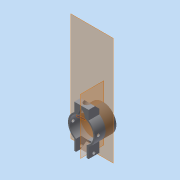
# Autodesk Inventor part: 13_Opentrons_Autofocus_Objectivering_Laser_Cam
Saved by Autodesk Inventor 2019.4 (Build 234330000, 330)
## iProperties
Created: 2020-12-16
Part Number: 13_Opentrons_Autofocus_Objectivering_Laser_Cam
Material: Generic
Document SubType Name: Modeling
Designer: diederichbenedict
Density: 1 g/cm^3
Appearance: Default
Author: diederichbenedict
Autodesk Inventor part; units mm, degrees
ref_plane "YZ Plane" through (0, 0, 0) normal (1, 0, 0) x (0, 1, 0)
ref_plane "XZ Plane" through (0, 0, 0) normal (0, 1, 0) x (-1, 0, 0)
ref_plane "XY Plane" through (0, 0, 0) normal (0, 0, 1) x (1, 0, 0)
ref_plane "Work Plane1" through (0, 0, 0) normal (0, 0, 1) x (1, 0, 0)
sketch "Sketch1" plane through (0, 0, 0) normal (0, 0, 1) x (1, 0, 0)
  circle A0 centre (0.9353, 17.3993) radius 11 projected
  circle A1 centre (0.9353, 17.3993) radius 11.1
  circle A2 centre (0.9353, 17.3993) radius 12.5
  point P0 (0, 0)
  dimension "d0" = 22.2
  dimension "d1" = 25
  constraints: 2 centre point, 2 coincident
  measures "d0" diameter of A1
  measures "d1" diameter of A2
extrude "Extrusion1" add sketch "Sketch1" against normal blind 10 contours A2
sketch "Sketch2" plane through (0.9353, 17.3993, 0) normal (0, 0, 1) x (1, 0, 0)
  circle A0 centre (0, 0) radius 12.5 projected
  circle A1 centre (0, 0) radius 11 construction
  ellipse E0 centre (0, 9.932) end of major axis (3, 9.932) minor radius 1.7207 construction
  ellipse E1 centre (0, -15.992) end of major axis (-4.2, -15.992) minor radius 2.409 construction
  circle A2 centre (0, 0) radius 11.1 projected
  line L0 (-6.6479, 19.2015) -> (6.6479, 19.2015)
  line L1 (6.6479, 19.2015) -> (6.6479, 10.5856)
  line L2 (-6.6479, 10.5856) -> (-6.6479, 19.2015)
  line L3 (-6.6479, 19.2015) -> (9.489, 5.7592) construction
  line L4 (6.6479, 19.2015) -> (-6.2726, 8.4385) construction
  line L5 (9.489, 5.7592) -> (9.3718, 5.7592) construction
  line L6 (-7.0563, 8.4385) -> (-6.2726, 8.4385) construction
  line L7 (-6.6479, -20.4673) -> (6.6479, -20.4673)
  line L8 (6.6479, -20.4673) -> (6.6479, -10.5856)
  line L9 (-6.6479, -10.5856) -> (-6.6479, -20.4673)
  line L10 (-6.6479, -20.4673) -> (6.6479, -10.5856) construction
  line L11 (6.6479, -20.4673) -> (-6.6479, -10.5856) construction
  line L12 (3.3398, -10.5856) -> (2.9907, -10.5856)
  line L13 (-2.9907, -10.5856) -> (-3.3398, -10.5856)
  point P0 (-0.9353, -17.3993)
  point P1 (0, 13.6637)
  point P2 (0, -15.5265)
  constraints: 28 end point, 11 point on circle, 6 parallel, 2 collinear, 2 horizontal, 2 midpoint, 2 perpendicular, 2 point on line, 1 coincident, 2 other
extrude "Extrusion3" add sketch "Sketch2" along normal blind 10
ref_plane "Work Plane2" through (-0.8941, 25.9676, 8.5979) normal (0, -0.819152, 0.5735764) x (0.7925374, -0.3497803, -0.499538)
ref_plane "Work Plane3" through (0.9353, -3.0679, 0) normal (1, 0, 0) x (0, 0, -1)
sketch "Sketch3" plane through (0.9353, -3.0679, 0) normal (1, 0, 0) x (0, 0, -1)
  line L0 (-7.6942, -1.3824) -> (-0.3218, 3.7798) projected
  line L1 (-9.1586, -2.4078) -> (-0.3397, 3.7672)
  line L2 (-0.3397, 3.7672) -> (-9.6168, 17.0163)
  line L3 (-9.6168, 17.0163) -> (-18.4357, 10.8412)
  line L4 (-18.4357, 10.8412) -> (-9.1586, -2.4078)
  line L5 (-9.1586, -2.4078) -> (-0.3397, 3.7672)
  line L6 (-0.3397, 3.7672) -> (-9.1586, -2.4078)
  line L7 (-0.3218, 3.7798) -> (-1.4689, 5.4181) construction
  line L8 (-0.3218, 3.7798) -> (-1.4689, 5.4181) construction
  line L9 (-7.6942, -1.3824) -> (-8.8413, 0.2559) construction
  line L10 (-7.6942, -1.3824) -> (-8.8413, 0.2559) construction
  point P0 (0, 3.0679)
  constraints: 12 end point, 4 equal length, 2 coincident, 1 perpendicular, 1 point on line, 5 other
extrude "Extrusion4" cut sketch "Sketch3" along normal mid plane 10
sketch "Sketch4" plane through (-0.8941, 25.9676, 8.5979) normal (0, -0.819152, 0.5735764) x (0.7925374, -0.3497803, -0.499538)
  circle A0 centre (0, 3) radius 3 projected
  circle A1 centre (0, 3) radius 3.15
  point P0 (14.0866, -16.841)
  dimension "d11" = 6.3
  constraints: 1 centre point, 1 coincident
  measures "d11" diameter of A1
extrude "Extrusion5" cut sketch "Sketch4" against normal through all contours A0 | A1
chamfer "Chamfer1" distance 4 angle 45 1 edges at (0.9353, 36.6008, 0)
sketch "Sketch5" plane through (0.9353, -3.0679, 0) normal (1, 0, 0) x (0, 0, -1)
  line L0 (10, 7.9673) -> (10, 32.9673) projected
  line L1 (0, 9.8817) -> (0, 9.8817) projected
  line L2 (0, 9.8817) -> (-10, 9.8817) projected
  line L3 (-10, 31.0529) -> (-10, 9.8817) projected
  line L4 (0, 31.0529) -> (-10, 31.0529) projected
  line L5 (0, 31.0529) -> (0, 31.0529) projected
  line L6 (0, 31.0529) -> (-10, 31.0529) projected
  line L7 (-10, 9.8817) -> (-10, 31.0529) projected
  line L8 (0, 9.8817) -> (-10, 9.8817) projected
  circle A0 centre (-6.4895, 20.4673) radius 1.45
  point P0 (0, 3.0679)
  dimension "d17" = 2.9
  constraints: 1 centre point
  measures "d17" diameter of A0
extrude "Extrusion6" cut sketch "Sketch5" along normal through all both and the other way through all
sketch "Sketch6" plane through (-5.7126, -3.0679, 0) normal (-1, 0, 0) x (0, 0, 1)
  line L0 (7.6942, -1.3824) -> (0.3218, 3.7798) projected
  line L1 (7.6942, -1.3824) -> (0.3218, 3.7798) projected
  line L2 (7.6942, -1.3824) -> (8.8413, 0.2559) projected
  line L3 (1.4689, 5.4181) -> (8.8413, 0.2559) projected
  line L4 (0.3218, 3.7798) -> (1.4689, 5.4181) projected
  circle A0 centre (4.8882, 2.4558) radius 1.45
  point P0 (0, 3.0679)
  dimension "d20" = 2.9
  constraints: 1 centre point
  measures "d20" diameter of A0
extrude "Extrusion7" cut sketch "Sketch6" against normal through all contours A0 L3 | L3 A0
pattern_circular "Circular Pattern1" count 2 over 30 about axis through (0.9353, 17.3993, 0) along (0, 0, -1) of "Extrusion6"
pattern_circular "Circular Pattern2" count 2 over 30 about axis through (0.9353, 17.3993, 0) along (0, 0, 1) of "Extrusion6"
body "Solid1"
